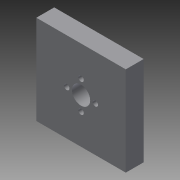
# Autodesk Inventor part: ACMENUTgen
Saved by Autodesk Inventor 2014 (Build 180170000, 170)
## iProperties
Created: 2015-11-30
Part Number: ACMENUTgen
Material: Generic
Document SubType Name: Modeling
Designer: cruiser
Density: 1 g/cm^3
Appearance: Default
Author: cruiser
Autodesk Inventor part; units mm, degrees
ref_plane "YZ Plane" through (0, 0, 0) normal (1, 0, 0) x (0, 1, 0)
ref_plane "XZ Plane" through (0, 0, 0) normal (0, 1, 0) x (-1, 0, 0)
ref_plane "XY Plane" through (0, 0, 0) normal (0, 0, 1) x (1, 0, 0)
sketch "Sketch1" plane through (0, 0, 0) normal (0, 1, 0) x (-1, 0, 0)
  line L0 (25, -25) -> (-25, -25)
  line L1 (-25, -25) -> (-25, 25)
  line L2 (-25, 25) -> (25, 25)
  line L3 (25, 25) -> (25, -25)
  line L4 (25, -25) -> (-25, 25) construction
  line L5 (-25, -25) -> (25, 25) construction
  point P0 (0, 0)
  dimension "d0" = 50
  dimension "d1" = 50
  constraints: 12 end point, 2 midpoint, 2 parallel, 1 horizontal, 1 perpendicular
  measures "d0" distance of L1.end L2.end
  measures "d1" distance of L0.end L1.end
extrude "Extrusion1" add sketch "Sketch1" along normal blind 10
sketch "Sketch2" plane through (0, 10, 0) normal (0, 1, 0) x (1, 0, 0)
  line L0 (25, -25) -> (25, 25) projected
  line L1 (0, 0) -> (0, 8)
  circle A0 centre (0, 8) radius 1.5
  circle A1 centre (0, 0) radius 5.1
  circle A2 centre (-8, 0) radius 1.5
  circle A3 centre (0, -8) radius 1.5
  circle A4 centre (8, 0) radius 1.5
  dimension "d4" = 8
  dimension "screw_hole" = 3
  dimension "center_hole" = 10.2
  dimension "d9" = 360
  constraints: 5 centre point, 2 coincident, 2 end point, 1 parallel, 9 other
  measures "d4" distance of L1.start L1.end
  measures "screw_hole" diameter of A0
  measures "center_hole" diameter of A1
extrude "Extrusion2" cut sketch "Sketch2" against normal up to next
body "Solid1"
